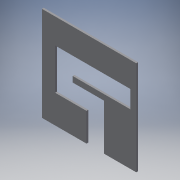
# Autodesk Inventor part: Plaque vois
Saved by Autodesk Inventor 2017 (Build 210142000, 142)
## iProperties
Part Number: Plaque vois
Material: Générique
Document SubType Name: Modeling
Designer: Thomas
Density: 1 g/cm^3
Appearance: Par défaut
Author: Thomas
Autodesk Inventor part; units mm, degrees
ref_plane "YZ Plane" through (0, 0, 0) normal (1, 0, 0) x (0, 1, 0)
ref_plane "XZ Plane" through (0, 0, 0) normal (0, 1, 0) x (-1, 0, 0)
ref_plane "XY Plane" through (0, 0, 0) normal (0, 0, 1) x (1, 0, 0)
sketch "Esquisse1" plane through (0, 0, 0) normal (0, 1, 0) x (-1, 0, 0)
  line L0 (0, 0) -> (300, 0)
  line L1 (300, 0) -> (300, -300)
  line L2 (300, -300) -> (0, -300)
  line L3 (0, -300) -> (0, 0)
  line L4 (158.1666, -300) -> (158.1666, -290)
  line L5 (158.1666, -290) -> (158.1666, -210)
  line L6 (158.1666, -210) -> (258.1666, -210)
  line L7 (258.1666, -210) -> (258.1666, -159)
  line L8 (202.1666, -154) -> (102.1666, -154)
  line L9 (158.1666, -300) -> (102.1666, -300)
  line L10 (102.1666, -300) -> (102.1666, -154)
  line L11 (202.1666, -136) -> (102.1666, -136)
  line L12 (215.9662, -80) -> (258.1666, -80)
  line L13 (258.1666, -80) -> (258.1666, -159)
  line L14 (215.9662, -80) -> (102.1666, -80)
  line L15 (202.1666, -136) -> (202.1666, -154)
  line L16 (102.1666, -136) -> (18.7834, -136)
  line L17 (18.7834, -136) -> (18.7834, -80)
  line L18 (18.7834, -80) -> (102.1666, -80)
  dimension "d0" = 300
  dimension "d1" = 300
  dimension "d4" = 100
  dimension "d7" = 56
  dimension "d13" = 146
  dimension "d14" = 100
  dimension "d15" = 130
  dimension "d17" = 56
  dimension "d18" = 90
  constraints: 38 end point, 9 perpendicular, 3 horizontal, 3 point on line, 2 parallel, 1 vertical
  measures "d0" distance of L1.end L2.end
  measures "d1" distance of L0.end L1.end
  measures "d4" distance of L5.end L6.end
  measures "d7" distance of L4.start L9.end
  measures "d13" distance of L9.end L8.end
  measures "d14" distance of L8.start L8.end
  measures "d15" distance between parallel lines of L6 L12
  measures "d17" distance between parallel lines of L11 L14
  measures "d18" distance between parallel lines of L9 L6
extrude "Extrusion2" add sketch "Esquisse1" along normal blind 6 contours L0 L1 L2 L4 L5 L6 L7 L13 L12 L14 L18 L17 L16 L11 L15 L8 L10 L3
